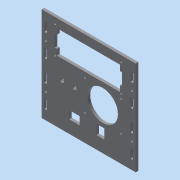
# Autodesk Inventor part: open reflow box
Saved by Autodesk Inventor 2013 (Build 170138000, 138)
## iProperties
Created: 2012-12-28
Part Number: open reflow box
Material: Generic
Document SubType Name: Modeling
Designer: Administrator
Density: 1 g/cm^3
Author: Administrator
Autodesk Inventor part; units mm, degrees
ref_plane "YZ Plane" through (0, 0, 0) normal (1, 0, 0) x (0, 1, 0)
ref_plane "XZ Plane" through (0, 0, 0) normal (0, 1, 0) x (-1, 0, 0)
ref_plane "XY Plane" through (0, 0, 0) normal (0, 0, 1) x (1, 0, 0)
sketch "Sketch1" plane through (0, 0, 0) normal (0, 0, 1) x (1, 0, 0)
  line L0 (-51.5546, 67.657) -> (55.1254, 67.657)
  line L1 (55.1254, 67.657) -> (55.1254, -39.023)
  line L2 (55.1254, -39.023) -> (-51.5546, -39.023)
  line L3 (-51.5546, -39.023) -> (-51.5546, 67.657)
  dimension "d0" = 106.68
  dimension "d2" = 106.68
  constraints: 8 end point, 2 parallel, 1 horizontal, 1 perpendicular
  measures "d0" distance of L2.end L0.start
  measures "d2" distance of L0.start L0.end
extrude "Extrusion1" add sketch "Sketch1" against normal blind 3
sketch "LCD Cut Out" plane through (0, 0, 0) normal (0, 0, 1) x (1, 0, 0)
  circle A0 centre (-36.5621, 61.0277) radius 1.25
  circle A1 centre (-36.5621, 30.0277) radius 1.25
  circle A2 centre (38.4379, 61.0277) radius 1.25
  circle A3 centre (38.4379, 30.0277) radius 1.25
  line L0 (-34.1482, 57.6923) -> (37.1518, 57.6923)
  line L1 (37.1518, 57.6923) -> (37.1518, 30.8923)
  line L2 (37.1518, 30.8923) -> (-34.1482, 30.8923)
  line L3 (-34.1482, 30.8923) -> (-34.1482, 57.6923)
  line L4 (37.1196, 51.3389) -> (39.6196, 51.3389)
  line L5 (39.6196, 51.3389) -> (39.6196, 37.5389)
  line L6 (39.6196, 37.5389) -> (37.1196, 37.5389)
  line L7 (37.1196, 37.5389) -> (37.1196, 51.3389)
  line L8 (-36.6336, 51.3389) -> (-34.1336, 51.3389)
  line L9 (-34.1336, 51.3389) -> (-34.1336, 37.5389)
  line L10 (-34.1336, 37.5389) -> (-36.6336, 37.5389)
  line L11 (-36.6336, 37.5389) -> (-36.6336, 51.3389)
  point P0 (0, 0)
  dimension "d96" = 76.2532
  constraints: 24 end point, 6 parallel, 4 centre point, 3 horizontal, 3 perpendicular
  measures "d96" distance between parallel lines of L5 L11
sketch "Sketch9" plane through (0, 0, 0) normal (0, 0, 1) x (1, 0, 0)
  circle A0 centre (-14.4313, 9.525) radius 2.4
  circle A1 centre (-28.575, 9.525) radius 2.4
  circle A2 centre (17.7335, 7.9375) radius 17.2
  circle A3 centre (-2.8375, 25.1375) radius 1.25
  circle A4 centre (38.1, 25.1375) radius 1.25
  circle A5 centre (38.1, -9.2625) radius 1.25
  circle A6 centre (-2.8375, -9.2625) radius 1.25
  line L0 (-20.4313, -15.698) -> (-8.4313, -15.698)
  line L1 (-8.4313, -15.698) -> (-8.4313, -24.698)
  line L2 (-8.4313, -24.698) -> (-20.4313, -24.698)
  line L3 (-20.4313, -24.698) -> (-20.4313, -15.698)
  line L4 (10.5687, -13.698) -> (19.5687, -13.698)
  line L5 (19.5687, -13.698) -> (19.5687, -24.698)
  line L6 (19.5687, -24.698) -> (10.5687, -24.698)
  line L7 (10.5687, -24.698) -> (10.5687, -13.698)
  line L8 (-51.5546, 67.657) -> (55.1254, 67.657) projected
  line L9 (55.1254, -39.023) -> (-51.5546, -39.023) projected
  line L10 (55.1254, 67.657) -> (55.1254, -39.023) projected
  circle A7 centre (-47.0546, 39.257) radius 1.525
  circle A8 centre (-47.0546, -10.623) radius 1.525
  circle A9 centre (50.6254, 39.257) radius 1.525
  circle A10 centre (50.6254, -10.623) radius 1.525
  line L11 (-48.6128, 57.182) -> (-45.5128, 57.182)
  line L12 (-45.5128, 57.182) -> (-45.5128, 47.082)
  line L13 (-45.5128, 47.082) -> (-48.6128, 47.082)
  line L14 (-48.6128, 47.082) -> (-48.6128, 57.182)
  line L15 (-45.5506, 31.432) -> (-48.6506, 31.432)
  line L16 (-48.6506, 31.432) -> (-48.6506, 21.332)
  line L17 (-48.6506, 21.332) -> (-45.5506, 21.332)
  line L18 (-45.5506, 21.332) -> (-45.5506, 31.432)
  line L19 (-45.5506, -2.798) -> (-48.6506, -2.798)
  line L20 (-48.6506, -2.798) -> (-48.6506, 7.302)
  line L21 (-48.6506, 7.302) -> (-45.5506, 7.302)
  line L22 (-45.5506, 7.302) -> (-45.5506, -2.798)
  line L23 (-45.5506, -18.448) -> (-48.6506, -18.448)
  line L24 (-48.6506, -18.448) -> (-48.6506, -28.548)
  line L25 (-48.6506, -28.548) -> (-45.5506, -28.548)
  line L26 (-45.5506, -28.548) -> (-45.5506, -18.448)
  line L27 (52.0999, 7.3659) -> (48.9999, 7.3659)
  line L28 (48.9999, 7.3659) -> (48.9999, -2.7341)
  line L29 (48.9999, -2.7341) -> (52.0999, -2.7341)
  line L30 (52.0999, -2.7341) -> (52.0999, 7.3659)
  line L31 (52.1638, -18.4611) -> (49.0638, -18.4611)
  line L32 (49.0638, -18.4611) -> (49.0638, -28.5611)
  line L33 (49.0638, -28.5611) -> (52.1638, -28.5611)
  line L34 (52.1638, -28.5611) -> (52.1638, -18.4611)
  line L35 (52.2687, 46.9823) -> (49.1687, 46.9823)
  line L36 (49.1687, 46.9823) -> (49.1687, 57.0823)
  line L37 (49.1687, 57.0823) -> (52.2687, 57.0823)
  line L38 (52.2687, 57.0823) -> (52.2687, 46.9823)
  line L39 (52.2687, 31.4608) -> (49.1687, 31.4608)
  line L40 (49.1687, 31.4608) -> (49.1687, 21.3608)
  line L41 (49.1687, 21.3608) -> (52.2687, 21.3608)
  line L42 (52.2687, 21.3608) -> (52.2687, 31.4608)
  point P0 (0, 0)
  dimension "d56" = 4.8
  dimension "d57" = 4.8
  dimension "d60" = 34.4
  dimension "d62" = 2.5
  dimension "d63" = 2.5
  dimension "d64" = 2.5
  dimension "d65" = 2.5
  dimension "d66" = 12
  dimension "d67" = 9
  dimension "d69" = 9
  dimension "d70" = 11
  dimension "d72" = 40
  dimension "d88" = 3.05
  dimension "d89" = 28.4
  dimension "d91" = 3.05
  dimension "d92" = 28.4
  dimension "d93" = 3.05
  dimension "d95" = 3.05
  dimension "d98" = 3.1
  dimension "d99" = 10.1
  dimension "d100" = 3.1
  dimension "d101" = 10.1
  dimension "d102" = 6.3
  dimension "d103" = 6.3
  dimension "d104" = 3.1
  dimension "d105" = 10.1
  dimension "d106" = 3.1
  dimension "d107" = 10.1
  dimension "d108" = 6.3
  dimension "d109" = 6.3
  dimension "d110" = 3.1
  dimension "d111" = 10.1
  dimension "d112" = 3.1
  dimension "d113" = 10.1
  dimension "d117" = 4.5
  dimension "d120" = 3.1
  dimension "d121" = 10.1
  dimension "d122" = 3.1
  dimension "d123" = 10.1
  dimension "d126" = 14.325
  dimension "d127" = 14.325
  constraints: 80 end point, 20 parallel, 11 centre point, 10 horizontal, 10 perpendicular
  measures "d56" diameter of A0
  measures "d57" diameter of A1
  measures "d60" diameter of A2
  measures "d62" diameter of A3
  measures "d63" diameter of A4
  measures "d64" diameter of A5
  measures "d65" diameter of A6
  measures "d66" distance of L0.start L0.end
  measures "d67" distance of L1.end L0.end
  measures "d69" distance of L4.start L4.end
  measures "d70" distance of L4.end L5.end
  measures "d72" distance between parallel lines of L5 L3
  measures "d88" diameter of A7
  measures "d89" distance from line of L8 A7.centre
  measures "d91" diameter of A8
  measures "d92" distance from line of L9 A8.centre
  measures "d93" diameter of A9
  measures "d95" diameter of A10
  measures "d98" distance of L12.end L13.end
  measures "d99" distance of L11.end L12.end
  measures "d100" distance of L17.end L16.end
  measures "d101" distance of L16.end L15.end
  measures "d102" distance edge to line of A7 L13
  measures "d103" distance edge to line of A7 L15
  measures "d104" distance of L20.end L21.end
  measures "d105" distance of L19.end L20.end
  measures "d106" distance of L25.end L24.end
  measures "d107" distance of L24.end L23.end
  measures "d108" distance edge to line of A8 L23
  measures "d109" distance edge to line of A8 L19
  measures "d110" distance of L29.end L28.end
  measures "d111" distance of L28.end L27.end
  measures "d112" distance of L33.end L32.end
  measures "d113" distance of L32.end L31.end
  measures "d117" distance from line of L10 A10.centre
  measures "d120" distance of L36.end L37.end
  measures "d121" distance of L35.end L36.end
  measures "d122" distance of L41.end L40.end
  measures "d123" distance of L40.end L39.end
  measures "d126" distance between parallel lines of L9 L2
  measures "d127" distance between parallel lines of L9 L6
extrude "Extrusion4" cut sketch "Sketch9" against normal blind 28.4
extrude "Extrusion5" cut sketch "LCD Cut Out" against normal blind 3
equation "\"d75\" = d89"
body "Solid1"
